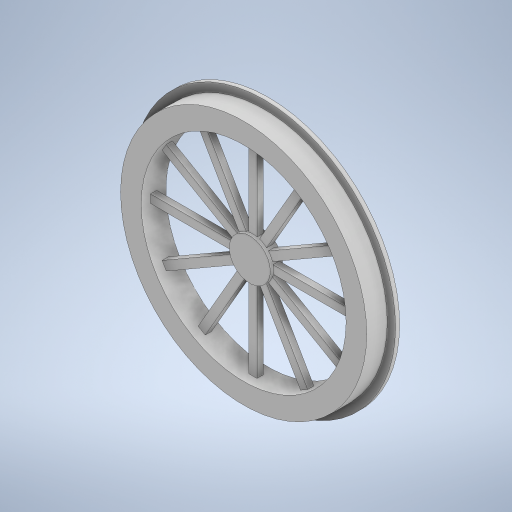
# Autodesk Inventor part: wheel
Saved by Autodesk Inventor 2023 (Build 270158000, 158)
## iProperties
Created: 2024-12-31
Part Number: wheel
Material: Generic
Document SubType Name: Modeling
Designer: Peter
Density: 1 g/cm^3
Appearance: Default
Author: Peter
Autodesk Inventor part; units mm, degrees
ref_plane "YZ Plane" through (0, 0, 0) normal (1, 0, 0) x (0, 1, 0)
ref_plane "XZ Plane" through (0, 0, 0) normal (0, 1, 0) x (-1, 0, 0)
ref_plane "XY Plane" through (0, 0, 0) normal (0, 0, 1) x (1, 0, 0)
sketch "Sketch1" plane through (0, 0, 0) normal (0, 0, 1) x (1, 0, 0)
  circle A0 centre (0, 0) radius 127
  dimension "d0" = 254
  constraints: 1 centre point, 1 coincident
  measures "d0" diameter of A0
extrude "Extrusion1" add sketch "Sketch1" along normal mid plane 76.2
sketch "Sketch2" plane through (0, 0, 0) normal (0, 0, 1) x (1, 0, 0)
  circle A0 centre (0, 0) radius 127 construction
  line L0 (-25.4, 124.4341) -> (25.4, 124.4341)
  line L1 (25.4, 124.4341) -> (25.4, 632.4341)
  line L2 (25.4, 632.4341) -> (-25.4, 632.4341)
  line L3 (-25.4, 632.4341) -> (-25.4, 124.4341)
  dimension "d3" = 50.8
  dimension "d4" = 508
  constraints: 8 end point, 2 parallel, 2 point on circle, 1 horizontal, 1 perpendicular
  measures "d3" distance of L1.end L2.end
  measures "d4" distance of L2.end L0.start
extrude "Extrusion2" add sketch "Sketch2" along normal mid plane 38.1
pattern_circular "Circular Pattern1" count 12 over 360 about axis through (0, 0, -10) along (0, 0, 1) of "Extrusion2"
sketch "Sketch3" plane through (0, 0, 0) normal (0, 0, 1) x (1, 0, 0)
  circle A0 centre (0, 0) radius 632.4341
  line L0 (25.4, 632.4341) -> (-25.4, 632.4341) projected
  arc A1 (-95.0631, 84.2141) -> (-120.4631, 40.22) centre (0, 0) ccw projected
  circle A2 centre (0, 0) radius 759.4341
  point P0 (0, 632.4341)
  dimension "d10" = 127
  constraints: 2 coincident, 1 centre point, 1 midpoint, 1 vertical alignment, 2 other
extrude "Extrusion3" add sketch "Sketch3" along normal mid plane 152.4
sketch "Sketch5" plane through (0, 0, -76.2) normal (0, 0, -1) x (-1, 0, 0)
  circle A0 centre (0, 0) radius 810.2341
  circle A1 centre (0, 0) radius 759.4341 projected
  circle A2 centre (0, 0) radius 759.4341
  dimension "d13" = 50.8
  constraints: 2 centre point, 2 coincident, 1 concentric
  measures "d13" radial gap between concentric circles of A1 A0
extrude "Extrusion4" add sketch "Sketch5" against normal blind 25.4
body "Solid1"
